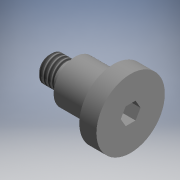
# Autodesk Inventor part: DBTS3-4.5-3-LTC
Saved by Autodesk Inventor 2017.3 (Build 213256000, 256)
## iProperties
Part Number: DBTS3-4.5-3-LTC
Material: Generic
Catalog Web Link: www.cadenas.de
Description: DBTB, DBTM, DBTS-Stepped Bolts - Low Head Type
Vendor: MISUMI
Document SubType Name: Modeling
Designer: partserver
Manufacturer: MISUMI
Mass: 0.202149 g
Surface Area: 2.62285 cm^2
Volume: 0.202149 cm^3
Density: 1 g/cm^3
Appearance: PSOLRGB-175-175-175
Category: PARTsolutions
Company: MISUMI
Title: DBTS3-4.5-3-LTC
Author: Cadenas PARTsolutions
Comments: Stepped Bolts - Low Head Type
PSOL_IDENT_0: {$CADENAS_DATA\23d-libs\misumi\metric\27_screws_nuts\dbtb.prj},208 {VTYP=3D},{NB=DBTS3-4.5-3-LTC},{L
PSOL_IDENT_1: INA=DBTS3-4.5-3-LTC},{NN=DBTB, DBTM, DBTS},{DATE=03.06.2021 03:35:29},{GEOMDATE=06.03.2020 06:09:28}
PSOL_IDENT_2: ,{VERSION=},{LINEID=10},{WBVAR=MAT,ST,ALT1,L,F,ALT2,ALT3},{WBNUMERIC=L,F}  {NB=DBTS3-4.5-3-LTC},{LIN
PSOL_IDENT_3: A=DBTS3-4.5-3-LTC},{KT=DUMMY},{PN=DBTS3-4.5-3-LTC},{TYPE=DBTS},{MAT=2},{ST=0},{ST0='0','-'},{M=3},{A
PSOL_IDENT_4: LT1=-LTC},{L=4.5},{F=3},{FA=(2:7/1)},{E=2.0},{D=5},{A=8},{B=2.0},{LL=1.0},{HH1=2.0},{P=0.5},{ALT2=},
PSOL_IDENT_5: {GG=0.0},{FF=0.0},{LINC=[3:20/0.1] },{ALT3=},{TOL=0/-0.2}
NB: DBTS3-4.5-3-LTC
NN: DBTB, DBTM, DBTS
NT: Stepped Bolts - Low Head Type
NBSYN: $PN.
LINA: DBTS3-4.5-3-LTC
CATALOG: Misumi
PN: DBTS3-4.5-3-LTC
MAT: 303 Stainless Steel
ST: -
M: 3
ALT1: with LTC (L Dimension Increment)
L: 4.5
F: 3
E: 2
D: 5
A: 8
B: 2
LL: 1
HH1: 2
ALT2: w/o PC (Relief on M)
ALT3: w/o DHC (Shaft Diameter Tolerance)
TOL: 0/-0.2
SUPPLIER: MISUMI
ARTICLENO: DBTS3-4.5-3-LTC
BOMINFO: DBTS3-4.5-3-LTC
CREATOR: CADENAS GmbH
Autodesk Inventor part; units mm, degrees
ref_plane "YZ Plane" through (0, 0, 0) normal (1, 0, 0) x (0, 1, 0)
ref_plane "XZ Plane" through (0, 0, 0) normal (0, 1, 0) x (-1, 0, 0)
ref_plane "XY Plane" through (0, 0, 0) normal (0, 0, 1) x (1, 0, 0)
sketch "Sketch_1" plane through (0, 0, 0) normal (0, 0, 1) x (1, 0, 0)
  line L0 (4.5, 0) -> (-2, 0)
  line L1 (-2, 0) -> (-2, 4)
  line L2 (-2, 4) -> (0, 4)
  line L3 (0, 4) -> (0, 2.5)
  line L4 (0, 2.5) -> (4.5, 2.5)
  line L5 (4.5, 2.5) -> (4.5, 0)
  line L6 (4.5, 0) -> (-2, 0)
  constraints: 14 end point
revolve "Revolution1" add sketch "Sketch_1" angle 360 about axis through (4.5, 0, 0) along (1, 0, 0)
sketch "Sketch2" plane through (-2, 0, 0) normal (-1, 0, 0) x (0, 0, 1)
  point P0 (0, 0)
hole "Hole1" at (-2, 0, 0) direction (1, 0, 0) diameter 2 depth 2 tip angle 120
sketch "Sketch_3" plane through (-2, 0, 0) normal (1, 0, 0) x (0, 0, -1)
  line L0 (-1, -0.5774) -> (0, -1.1547)
  line L1 (0, -1.1547) -> (1, -0.5774)
  line L2 (1, -0.5774) -> (1, 0.5774)
  line L3 (1, 0.5774) -> (0, 1.1547)
  line L4 (0, 1.1547) -> (-1, 0.5774)
  line L5 (-1, 0.5774) -> (-1, -0.5774)
  constraints: 12 end point
extrude "Extrusion1" cut sketch "Sketch_3" along normal blind 2
sketch "Sketch_6" plane through (0, 0, 0) normal (0, 0, 1) x (1, 0, 0)
  line L0 (7.5, 0) -> (4.5, 0)
  line L1 (4.5, 0) -> (4.5, 1.5)
  line L2 (4.5, 1.5) -> (7.1935, 1.5)
  line L3 (7.1935, 1.5) -> (7.5, 1.1935)
  line L4 (7.5, 1.1935) -> (7.5, 0)
  line L5 (7.5, 0) -> (4.5, 0)
  constraints: 12 end point
revolve "Revolution2" add sketch "Sketch_6" angle 360 about axis through (7.5, 0, 0) along (1, 0, 0)
thread "Thread1" size "M3x0.5" class "6g" standard "ISO Metric profile" length 1.6935
body "Solid1"
